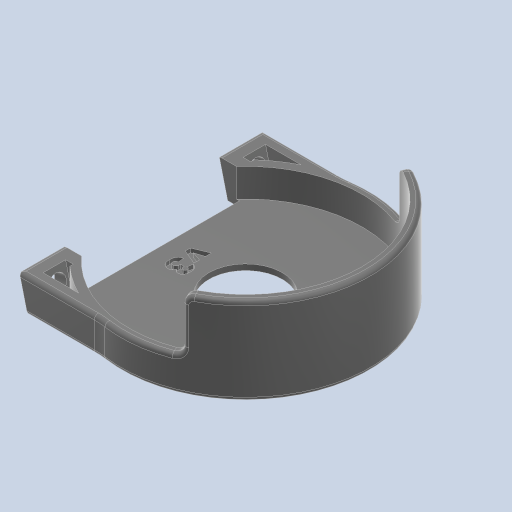
# Autodesk Inventor part: wb_holder_outside_03a
Saved by Autodesk Inventor 2024.4 (Build 284460000, 460)
## iProperties
Created: 2026-05-05
Part Number: wb_holder_outside_03a
Material: PLA Black
Document SubType Name: Modeling
Designer: tooles01
Density: 1.06 g/cm^3
Appearance: Smooth - White(2)
Author: tooles01
Autodesk Inventor part; units mm, degrees
ref_plane "YZ Plane" through (0, 0, 0) normal (1, 0, 0) x (0, 1, 0)
ref_plane "XZ Plane" through (0, 0, 0) normal (0, 1, 0) x (-1, 0, 0)
ref_plane "XY Plane" through (0, 0, 0) normal (0, 0, 1) x (1, 0, 0)
sketch "Sketch1: base" plane through (0, 0, 0) normal (0, 1, 0) x (-1, 0, 0)
  circle A0 centre (0, 0) radius 28.5
  circle A1 centre (0, 0) radius 30.5
  circle A2 centre (0, 0) radius 9
  line L0 (30.5, -16) -> (30.5, 21.2627) construction
  line L1 (28.5, -16) -> (28.5, 21.2627) construction
  line L2 (20.5, -22.5832) -> (20.5, 22.5832)
  point P0 (20.5, -19.799)
  point P1 (20.5, 19.799)
  dimension "d0" = 57
  dimension "d6" = 18
  dimension "d1" = 2
  dimension "d83" = 10
  constraints: 6 end point, 3 centre point, 3 coincident, 3 vertical, 2 point on circle, 2 tangent, 1 horizontal alignment, 1 parallel
  measures "d0" diameter of A0
  measures "d6" diameter of A2
  measures "d1" radial gap between concentric circles of A0 A1
  measures "d83" distance between parallel lines of L0 L2
extrude "Ex1: base" add sketch "Sketch1: base" against normal blind 1.4 contours L2 A0 | A0 L2 A1 | A2 picked at (16.6667, 0) picked at (18.656, 22.2117)
extrude "Ex2: outer edge" add sketch "Sketch1: base" along normal blind 18 contours A0 L2 A1 picked at (18.656, 22.2117)
extrude "Ex3: hole for spout" cut sketch "Sketch1: base" against normal through all contours A2
sketch "Sketch2: connect to cage wall" plane through (0, 0, 0) normal (0, 0, 1) x (1, 0, 0)
  line L0 (-25.4354, 6.7624) -> (-22.5245, 7.4881)
  line L1 (-22.5245, 7.4881) -> (-20.5891, -0.2742)
  line L2 (-20.5891, -0.2742) -> (-23.5, -1)
  line L3 (-23.5, -1) -> (-25.4354, 6.7624)
  line L4 (-36.6, 0) -> (6.1, 0) construction
  line L5 (-30.5, 18) -> (-28.5, 18) construction
  line L6 (-28.5, 18) -> (-28.5, -1.4) construction
  line L7 (-28.5, -1.4) -> (-30.5, -1.4) construction
  line L8 (-30.5, -1.4) -> (-30.5, 18) construction
  point P0 (0, 0)
  point P1 (-30.5, 0)
  point P2 (-30.5, 0)
  point P3 (-30.5, 0)
  point P4 (-28.5, 0)
  point P5 (-28.5, 0)
  point P6 (-28.5, 0)
  dimension "d12" = 1.4
  dimension "d13" = 18
  dimension "d18" = 3
  dimension "d23" = 8
  dimension "d33" = 1
  dimension "d65" = 14
  dimension "d82" = 7
  constraints: 16 end point, 6 perpendicular, 2 point on line, 1 horizontal, 1 other
  measures "d12" distance from line of L7 point (-28.5, 0)
  measures "d13" distance from line of L5 point (-28.5, 0)
  measures "d18" distance of L0.start L0.end
  measures "d23" distance of L2.end L0.start
  measures "d65" angle to the sketch x axis of L2
  measures "d82" distance from line of L8 L2.end
extrude "Ex4: connect to cage wall" add sketch "Sketch2: connect to cage wall" along normal mid plane 60
sketch "Sketch3: heat-set inserts" plane through (-23.5, -1, -30) normal (-0.9702957, -0.2419219, 0) x (0, 0, 1)
  circle A0 centre (5.5, 4) radius 2.1
  circle A1 centre (54.5, 4) radius 2.1
  line L0 (30, 0) -> (30, 8) construction
  line L1 (0, 0) -> (0, 8) construction
  line L2 (60, 8) -> (60, 0) construction
  line L3 (0, 8) -> (60, 8) construction
  line L4 (60, 0) -> (0, 0) construction
  point P0 (30, -4.7149)
  point P1 (0, 4)
  dimension "m3_heat_set" = 4.2
  dimension "d20" = 5.5
  constraints: 2 centre point, 1 equal radius, 1 horizontal alignment, 1 midpoint, 1 other
  measures "m3_heat_set" diameter of A0
  measures "d20" distance from line of A0.centre L1
extrude "Ex5: heat-set inserts" cut sketch "Sketch3: heat-set inserts" against normal up to surface (3 mm away)
sketch "Sketch4: cut center of screw part" plane through (-23.5, -1, -30) normal (-0.9702957, -0.2419219, 0) x (0, 0, 1)
  circle A0 centre (54.5, 4) radius 2.1 projected
  circle A1 centre (5.5, 4) radius 2.1 projected
  line L0 (60, 0) -> (0, 0) projected
  line L1 (60, 8) -> (60, 0) projected
  line L2 (0, 8) -> (60, 8) projected
  line L3 (0, 0) -> (0, 8) projected
  line L4 (11, 0) -> (11, 8)
  line L5 (49, 0) -> (49, 8)
  line L6 (60, 0) -> (0, 0) projected
  point P0 (30, -4.7149)
  point P1 (11, 0)
  dimension "d25" = 5.5
  dimension "d27" = 5.5
  constraints: 4 end point, 4 point on line, 2 perpendicular
  measures "d25" distance from line of L4 A1.centre
  measures "d27" distance from line of L5 A0.centre
extrude "Ex6: cut center of screw part" cut sketch "Sketch4: cut center of screw part" against normal up to surface (3 mm away) contours L0 L4 L2 L5
sketch "Sketch6: extend back to circle" plane through (-25.4354, 6.7624, -30) normal (-0.9702957, -0.2419219, 0) x (0, 0, 1)
  line L0 (11, -8) -> (11, 0) projected
  line L1 (0, 0) -> (11, 0) projected
  line L2 (0, -8) -> (0, 0) projected
  line L3 (11, -8) -> (0, -8) projected
  circle A0 centre (5.5, -4) radius 2.1 projected
  line L4 (49, 0) -> (49, -8) projected
  line L5 (60, -8) -> (49, -8) projected
  line L6 (60, 0) -> (60, -8) projected
  line L7 (49, 0) -> (60, 0) projected
  circle A1 centre (54.5, -4) radius 2.1 projected
  line L8 (2.75, 0) -> (8.25, 0)
  line L9 (8.25, 0) -> (8.25, -8)
  line L10 (8.25, -8) -> (2.75, -8)
  line L11 (2.75, -8) -> (2.75, 0)
  line L12 (51.75, 0) -> (57.25, 0)
  line L13 (57.25, 0) -> (57.25, -8)
  line L14 (57.25, -8) -> (51.75, -8)
  line L15 (51.75, -8) -> (51.75, 0)
  line L16 (0, 0) -> (11, 0) projected
  line L17 (49, 0) -> (60, 0) projected
  point P0 (30, -12.7149)
  point P1 (51.75, 0)
  point P2 (8.25, 0)
  point P3 (2.75, -8)
  point P4 (2.75, 0)
  dimension "d67" = 2.75
  dimension "d68" = 2.75
  dimension "d69" = 2.75
  constraints: 16 end point, 5 collinear, 4 perpendicular
  measures "d67" distance between parallel lines of L0 L9
  measures "d68" distance between parallel lines of L6 L13
  measures "d69" distance between parallel lines of L2 L11
extrude "Ex7: extend back to circle" add sketch "Sketch6: extend back to circle" against normal up to surface contours L3 L9 L1 L0 | L3 L2 L1 L11 | L7 L15 L5 L4 | L7 L6 L5 L13 round surface about axis through (0, 0, 0) along (0, -1, 0) radius 30.5 far side no
sketch "Sketch9: for printing" plane through (0, 0, 30) normal (0, 0, 1) x (1, 0, 0)
  line L0 (-5.5, 3.4879) -> (-5.5, -1.4)
  line L1 (-5.5, -1.4) -> (-23.4003, -1.4)
  line L2 (-20.5, -1.4) -> (30.5, -1.4) projected
  line L3 (-23.4003, -1.4) -> (-23.5, -1)
  line L4 (-23.5, -1) -> (-5.5, 3.4879) projected
  line L5 (-25.4354, 6.7624) -> (-23.5, -1) construction
  point P0 (0, 0)
  constraints: 6 end point, 2 collinear, 1 perpendicular
extrude "Ex10: for printing-1R" add sketch "Sketch9: for printing" against normal up to surface (2.75 mm away)
extrude "Ex10: for printing-1L" add sketch "Sketch9: for printing" against normal up to surface (2.75 mm away) from surface at -8.25
extrude "Ex10: for printing-2R" add sketch "Sketch9: for printing" against normal up to surface (2.75 mm away) from surface at -49
extrude "Ex10: for printing-2L" add sketch "Sketch9: for printing" along normal up to surface (2.75 mm away) from surface at -60
sketch "Sketch10: for printing" plane through (-20.5891, -0.2742, -27.25) normal (0.2419219, -0.9702957, 0) x (0.9702957, 0.2419219, 0)
  line L0 (-3, 0) -> (0, 0) projected
  line L1 (0, 0) -> (0, 5.5) projected
  line L2 (0, 5.5) -> (-3, 5.5) projected
  line L3 (-3, 5.5) -> (-3, 0) projected
  line L4 (-3, 49) -> (0, 49) projected
  line L5 (0, 49) -> (0, 54.5) projected
  line L6 (0, 54.5) -> (-3, 54.5) projected
  line L7 (-3, 54.5) -> (-3, 49) projected
  point P0 (20.0439, 27.25)
extrude "Ex11: for printing" add sketch "Sketch10: for printing" along normal up to surface surface through (5, -1.4, 0) normal (0, 1, 0)
extrude "Ex8: clean the inside" cut sketch "Sketch1: base" against normal up to surface (18 mm away) from surface at 18 contours A0 L2 | L2 A0
sketch "Sketch11: slice the top" plane through (0, 0, 0) normal (0, 0, 1) x (1, 0, 0)
  line L0 (-25.4354, 30.1388) -> (30.5, 30.1388)
  line L1 (30.5, 30.1388) -> (30.5, 6.9188)
  line L2 (30.5, 6.9188) -> (-25.4354, 6.9188)
  line L3 (-25.4354, 6.9188) -> (-25.4354, 30.1388)
  line L4 (-23.9597, 0.8436) -> (-24.9757, 4.9188) projected
  line L5 (30.5, 30.1388) -> (-20, 18) construction
  line L6 (-25.4354, 6.7624) -> (-23.5, -1) construction
  point P0 (0, 0)
  dimension "d56" = 2
  constraints: 10 end point, 3 perpendicular, 1 horizontal, 1 vertical alignment
  measures "d56" distance from line of L2 L4.end
extrude "Ex: slice the top" cut sketch "Sketch11: slice the top" along normal through all both and the other way through all
sketch "Sketch12: raise the back" plane through (0, 0, 0) normal (0, 1, 0) x (-1, 0, 0)
  circle A0 centre (0, 0) radius 30.5 projected
  circle A1 centre (0, 0) radius 28.5 projected
  ellipse E0 centre (24.4677, 24.5) end of major axis (24.4677, 26.6) minor radius 0.508 construction
  ellipse E1 centre (24.4677, -24.5) end of major axis (24.4677, -22.4) minor radius 0.508 construction
  line L0 (25.4354, -30) -> (5.5, -30) construction
  line L1 (23.859, -19) -> (25.4354, -19) construction
  line L2 (25.4354, -19) -> (25.4354, -30) construction
  line L3 (25.4354, 19) -> (23.859, 19) construction
  line L4 (5.5, 30) -> (25.4354, 30) construction
  line L5 (25.4354, 30) -> (25.4354, 19) construction
  line L6 (-12.4917, -27.8246) -> (-11.6726, -26)
  line L7 (-12.4917, 27.8246) -> (-11.6726, 26)
  line L8 (21.121, 16.8197) -> (23.859, 19)
  line L9 (23.859, -19) -> (21.121, -16.8197)
  line L10 (42.7, 0) -> (-42.7, 0) construction
  arc A2 (21.121, -16.8197) -> (21.121, 16.8197) centre (0, 0) ccw
  line L11 (25.4354, -30) -> (25.4354, -19) construction
  line L12 (25.4354, 19) -> (25.4354, 30) construction
  point P0 (22.2944, -17.7541)
  point P1 (22.2944, 17.7541)
  dimension "d63" = 1.5
  dimension "d64" = 52
  constraints: 20 end point, 4 perpendicular, 4 point on circle, 1 centre point, 1 concentric, 14 other
  measures "d63" radial gap between concentric circles of A1 A2
  measures "d64" distance of L6.end L7.end
extrude "Ex16: raise the back" add sketch "Sketch12: raise the back" along normal blind 20 contours L7 A1 L6 A0
extrude "Ex17: slice the front" [suppressed]
fillet "Fillet1" radius 20 2 edges at (-5.5, 2.7594, 30) (-5.5, 2.7594, -30)
fillet "Fillet2" radius 2 4 edges at (12.0822, 6.9188, 26.9123) (12.0822, 6.9188, -26.9123) (12.0822, 20, 26.9123) (12.0822, 20, -26.9123)
fillet "Fillet3" radius 1 18 edges at (12.9351, 19.3089, -27.6212) (12.4917, 13.4594, -27.8246) (12.0485, 7.6141, -28.0194) (3.2803, 6.9188, -30.3231) (-5.6815, 6.9188, -30.0496) (-15.9483, 6.9188, -30) (12.9352, 19.3089, 27.6212) (12.4917, 13.4594, 27.8246) (12.0485, 7.6141, 28.0194) (3.2803, 6.9188, 30.3231) (-5.6815, 6.9188, 30.0496) (-15.9483, 6.9188, 30) (30.5, 20, 0) (-5.6815, -1.4, 30.0496) (-15.2445, -1.4, 30) (-5.6815, -1.4, -30.0496) (-15.2445, -1.4, -30) (30.5, -1.4, 0)
sketch "Sketch15" plane through (0, 0, 0) normal (0, 1, 0) x (-1, 0, 0)
  line L0 (12, -2) -> (12, 2) construction
  line L1 (12, 2) -> (16, 2) construction
  line L2 (16, 2) -> (16, -2) construction
  line L3 (16, -2) -> (12, -2) construction
  line L4 (12.8763, -4.4562) -> (12.8763, -3.0125)
  line L5 (12.8763, -3.0125) -> (15.1718, -2.3051)
  line L6 (15.1718, -2.3051) -> (12.8763, -1.5784)
  line L7 (12.8763, -1.5784) -> (12.8763, -0.1781)
  line L8 (12.8763, -0.1781) -> (16.5, -1.718)
  line L9 (16.5, -1.718) -> (16.5, -2.95)
  line L10 (16.5, -2.95) -> (12.8763, -4.4562)
  line L11 (12.9437, 1.4389) -> (12.7079, 0.1251)
  spline S0 degree 2 poles (12.7079, 0.1251) (12.0823, 0.2887) (11.4134, 1.2175) (11.4134, 2.0693) knots 0 0 0 1 2 2 2
  spline S1 degree 2 poles (11.4134, 2.0693) (11.4134, 3.051) (12.1449, 3.922) (12.6935, 3.922) knots 0 0 0 1 2 2 2
  spline S2 degree 2 poles (12.6935, 3.922) (13.0207, 3.922) (13.5452, 3.5659) (13.7425, 3.205) knots 0 0 0 1 2 2 2
  spline S3 degree 2 poles (13.7425, 3.205) (13.8147, 3.4986) (13.911, 3.6526) knots 0 0 0 1 1 1
  spline S4 degree 2 poles (13.911, 3.6526) (14.065, 3.9028) (14.5654, 4.1771) (14.9119, 4.1771) knots 0 0 0 1 2 2 2
  spline S5 degree 2 poles (14.9119, 4.1771) (15.3499, 4.1771) (16.1535, 3.7199) (16.5866, 2.8633) (16.5866, 2.1607) knots 0 0 0 1 2 3 3 3
  spline S6 degree 2 poles (16.5866, 2.1607) (16.5866, 1.4822) (16.2642, 0.693) (15.6482, 0.1829) (15.1814, 0.0481) knots 0 0 0 1 2 3 3 3
  line L12 (15.1814, 0.0481) -> (14.9986, 1.4389)
  spline S7 degree 2 poles (14.9986, 1.4389) (15.4172, 1.5207) (15.7397, 1.8624) (15.7397, 2.127) knots 0 0 0 1 2 2 2
  spline S8 degree 2 poles (15.7397, 2.127) (15.7397, 2.4062) (15.3306, 2.7767) (14.9889, 2.7767) knots 0 0 0 1 2 2 2
  spline S9 degree 2 poles (14.9889, 2.7767) (14.6376, 2.7767) (14.2575, 2.4206) (14.2575, 2.1126) knots 0 0 0 1 2 2 2
  spline S10 degree 2 poles (14.2575, 2.1126) (14.2575, 1.949) (14.3393, 1.6651) knots 0 0 0 1 1 1
  line L13 (14.3393, 1.6651) -> (13.3431, 1.7372)
  spline S11 degree 2 poles (13.3431, 1.7372) (13.3624, 1.8527) (13.3624, 1.9153) knots 0 0 0 1 1 1
  spline S12 degree 2 poles (13.3624, 1.9153) (13.3624, 2.1896) (13.0159, 2.5553) (12.7753, 2.5553) knots 0 0 0 1 2 2 2
  spline S13 degree 2 poles (12.7753, 2.5553) (12.5491, 2.5553) (12.2748, 2.281) (12.2748, 2.0452) knots 0 0 0 1 2 2 2
  spline S14 degree 2 poles (12.2748, 2.0452) (12.2748, 1.7998) (12.5731, 1.4918) (12.9437, 1.4389) knots 0 0 0 1 2 2 2
  point P0 (0, 0)
  point P1 (12, 0)
  dimension "d77" = 4
  dimension "d78" = 12
  constraints: 1 horizontal, 1 horizontal alignment, 1 midpoint, 1 perpendicular, 2 other
  measures "d77" distance of L0.start L0.end
  measures "d78" distance from line of point (0, 0) L0
extrude "Ex20: text" cut sketch "Sketch15" against normal blind 1
equation "\"d12\" = d2"
equation "\"d13\" = d4"
equation "\"d25\" = d20"
equation "\"d27\" = d25"
equation "\"d68\" = d67"
equation "\"d2\" = 1.4"
equation "\"d4\" = 18"
body "Solid1"
